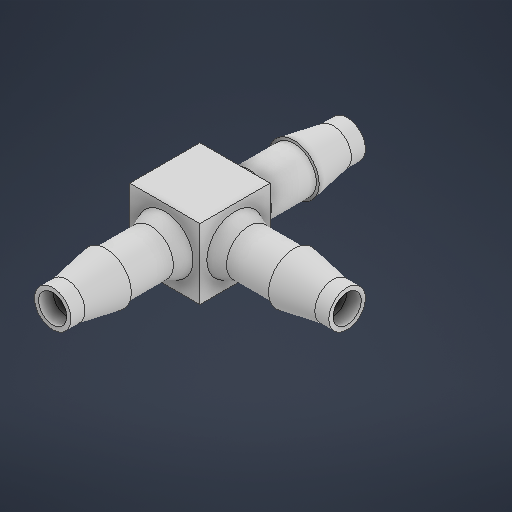
# Autodesk Inventor part: Adafruit_4662
Saved by Autodesk Inventor 2026.2 (Build 302298000, 298)
## iProperties
Created: 2026-02-03
Part Number: Adafruit_4662
Material: Generic
Document SubType Name: Modeling
Designer: vckot
Density: 1 g/cm^3
Appearance: Default
Author: vckot
Autodesk Inventor part; units mm, degrees
ref_plane "YZ Plane" through (0, 0, 0) normal (1, 0, 0) x (0, 1, 0)
ref_plane "XZ Plane" through (0, 0, 0) normal (0, 1, 0) x (-1, 0, 0)
ref_plane "XY Plane" through (0, 0, 0) normal (0, 0, 1) x (1, 0, 0)
sketch "Sketch1" plane through (0, 0, 0) normal (0, 0, 1) x (1, 0, 0)
  line L0 (-3.125, -3.125) -> (3.125, -3.125)
  line L1 (3.125, -3.125) -> (3.125, 3.125)
  line L2 (3.125, 3.125) -> (-3.125, 3.125)
  line L3 (-3.125, 3.125) -> (-3.125, -3.125)
  line L4 (-3.125, -3.125) -> (3.125, 3.125) construction
  line L5 (3.125, -3.125) -> (-3.125, 3.125) construction
  point P0 (0, 0)
  dimension "d0" = 6.25
  dimension "d1" = 6.25
  constraints: 12 end point, 2 midpoint, 2 parallel, 1 horizontal, 1 perpendicular
  measures "d0" distance of L2.end L1.end
  measures "d1" distance of L1.end L0.end
extrude "Extrusion1" add sketch "Sketch1" along normal mid plane 6.25
sketch "Sketch2" plane through (0, 0, 0) normal (1, 0, 0) x (0, 1, 0)
  line L0 (-3.125, 3.125) -> (3.125, 3.125) projected
  line L1 (2, 4.375) -> (2, 8.375)
  line L2 (2, 8.375) -> (2.25, 8.375)
  line L3 (2.25, 8.375) -> (1.625, 11.875)
  line L4 (0, 0) -> (0, 14.1963) construction
  line L5 (1.625, 11.875) -> (1.625, 13.125)
  line L6 (2, 4.375) -> (2.5, 3.125)
  line L7 (1.25, 13.125) -> (1.25, 11.8418)
  line L8 (1.25, 11.8418) -> (1.8021, 8.75)
  line L9 (1.8021, 8.75) -> (1.625, 8.75)
  line L10 (1.625, 8.75) -> (1.625, 4.3028)
  line L11 (1.625, 4.3028) -> (2.1518, 2.9857)
  line L12 (1.625, 13.125) -> (1.25, 13.125)
  point P0 (2.0961, 3.125)
  dimension "d4" = 4
  dimension "d5" = 4.5
  dimension "d6" = 3.25
  dimension "d7" = 10
  dimension "d8" = 1.25
  dimension "d9" = 3.5
  dimension "d11" = 5
  dimension "d12" = 1.25
  dimension "d13" = 2.5
  constraints: 24 end point, 3 vertical, 2 perpendicular, 1 horizontal, 1 point on line, 4 other
  measures "d4" diameter of L1 L4
  measures "d5" diameter of L2.end L4
  measures "d6" diameter of L5 L4
  measures "d7" distance from line of L0 L5.end
  measures "d8" distance of L3.end L5.end
  measures "d9" vertical distance of L2.end L3.end
  measures "d11" diameter of L6.end L4
  measures "d12" vertical distance of L1.start L6.end
  measures "d13" diameter of L7 L4
revolve "Revolution1" add sketch "Sketch2" angle 360 about axis through (0, 0, 0) along (0, 0, 1)
pattern_circular "Circular Pattern1" count 3 over 180 about axis through (0, -10, 0) along (0, 1, 0) of "Revolution1"
equation "\"d2\" = d1"
body "Solid1"
